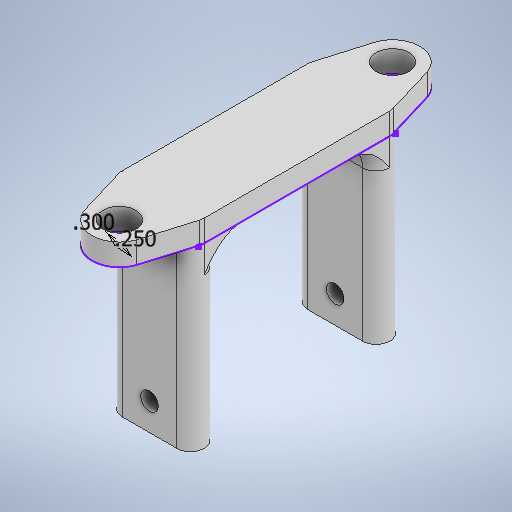
# Autodesk Inventor part: Latest_Odom
Saved by Autodesk Inventor 2025.1 (Build 291241020, 241B)
## iProperties
Created: 2024-11-18
Part Number: Latest_Odom
Material: Generic
Document SubType Name: Modeling
Designer: colli
Density: 1 g/cm^3
Appearance: Default
Author: colli
Autodesk Inventor part; units mm, degrees
ref_plane "YZ Plane" through (0, 0, 0) normal (1, 0, 0) x (0, 1, 0)
ref_plane "XZ Plane" through (0, 0, 0) normal (0, 1, 0) x (-1, 0, 0)
ref_plane "XY Plane" through (0, 0, 0) normal (0, 0, 1) x (1, 0, 0)
sketch "Sketch1" plane through (0, 0, 0) normal (0, 1, 0) x (-1, 0, 0)
  line L0 (1.8331, 41.275) -> (-1.8331, 41.275)
  line L1 (-1.8331, 41.275) -> (-3.6662, 38.1)
  line L2 (-3.6662, 38.1) -> (-1.8331, 34.925)
  line L3 (-1.8331, 34.925) -> (1.8331, 34.925)
  line L4 (1.8331, 34.925) -> (3.6662, 38.1)
  line L5 (3.6662, 38.1) -> (1.8331, 41.275)
  circle A0 centre (0, 38.1) radius 2.0955
  circle A1 centre (0, 38.1) radius 3.0353
  arc A2 (6.0168, 40.1299) -> (-6.0168, 40.1299) centre (0, 38.1) ccw
  line L6 (6.35, 24.765) -> (-6.35, 24.765)
  arc A3 (-6.35, 31.115) -> (-6.35, 24.765) centre (-6.35, 27.94) ccw
  arc A4 (6.35, 24.765) -> (6.35, 31.115) centre (6.35, 27.94) ccw
  line L7 (9.525, 27.94) -> (9.525, 19.812)
  line L8 (-9.525, 27.94) -> (-9.525, 19.812)
  circle A5 centre (0, 38.1) radius 3.81
  line L9 (-9.525, 19.812) -> (-9.525, 6.35)
  line L10 (9.525, 19.812) -> (9.525, 6.35)
  line L11 (0, 19.812) -> (0, -7.112) construction
  line L12 (0, 38.1) -> (0, 31.75)
  line L13 (9.525, -15.24) -> (9.525, 6.35)
  line L14 (-9.525, -15.24) -> (-9.525, 6.35)
  line L15 (6.35, 31.115) -> (-6.35, 31.115)
  line L16 (-6.0168, 40.1299) -> (-9.3918, 28.8501)
  line L17 (6.0168, 40.1299) -> (9.3918, 28.8501)
  line L18 (1.8331, -28.575) -> (-1.8331, -28.575)
  line L19 (-1.8331, -28.575) -> (-3.6662, -25.4)
  line L20 (-3.6662, -25.4) -> (-1.8331, -22.225)
  line L21 (-1.8331, -22.225) -> (1.8331, -22.225)
  line L22 (1.8331, -22.225) -> (3.6662, -25.4)
  line L23 (3.6662, -25.4) -> (1.8331, -28.575)
  circle A6 centre (0, -25.4) radius 2.0955
  circle A7 centre (0, -25.4) radius 3.0353
  arc A8 (-6.0168, -27.4299) -> (6.0168, -27.4299) centre (0, -25.4) ccw
  line L24 (6.35, -12.065) -> (-6.35, -12.065)
  arc A9 (-6.35, -12.065) -> (-6.35, -18.415) centre (-6.35, -15.24) ccw
  arc A10 (6.35, -18.415) -> (6.35, -12.065) centre (6.35, -15.24) ccw
  line L25 (9.525, -15.24) -> (9.525, -7.112)
  line L26 (-9.525, -15.24) -> (-9.525, -7.112)
  circle A11 centre (0, -25.4) radius 3.81
  line L27 (0, -25.4) -> (0, -19.05)
  line L28 (6.35, -18.415) -> (-6.35, -18.415)
  line L29 (-6.0168, -27.4299) -> (-9.3918, -16.1501)
  line L30 (6.0168, -27.4299) -> (9.3918, -16.1501)
  point P0 (0, 0)
  point P1 (9.525, 29.21)
  point P2 (-9.525, 29.21)
  point P3 (-9.525, -16.51)
  point P4 (9.525, -16.51)
  dimension "d35" = 7.62
  dimension "d91" = 6.35
  constraints: 64 end point, 8 centre point, 4 coincident, 4 point on circle, 1 horizontal, 1 vertical, 26 other
  measures "d35" diameter of A5
  measures "d91" distance of L12.start L12.end
extrude "Extrusion18" add sketch "Sketch1" along normal blind 5.08 contours L17 A4 L15 A3 L16 A2 | A4 L6 A3 L15 | L7 L10 L13 A10 L24 A9 L14 L9 L8 A3 L6 A4 | A10 L28 A9 L24 | L30 A8 L29 A9 L28 A10
extrude "Extrusion19" add sketch "Sketch1" against normal blind 41.275 contours A4 L6 A3 L15 | A10 L28 A9 L24
fillet "Fillet5" radius 6.35 6 edges at (-8.5951, 0, 25.6949) (8.5951, 0, 25.6949) (0, 0, 24.765) (8.5951, 0, -12.9949) (-8.5951, 0, -12.9949) (0, 0, -12.065)
sketch "Sketch12" plane through (-6.35, 0, 31.115) normal (0, 0, 1) x (1, 0, 0)
  line L0 (12.7, -41.275) -> (0, -41.275) projected
  line L1 (6.35, -41.275) -> (6.35, -34.925)
  circle A0 centre (6.35, -34.925) radius 2.032
  point P0 (6.35, 0)
  dimension "d98" = 6.35
  dimension "d99" = 4.064
  constraints: 2 end point, 1 centre point, 1 coincident, 1 midpoint, 1 vertical
  measures "d98" distance of L1.start L1.end
  measures "d99" diameter of A0
extrude "Extrusion20" cut sketch "Sketch12" along normal through all both and the other way through all
body "Solid2"
